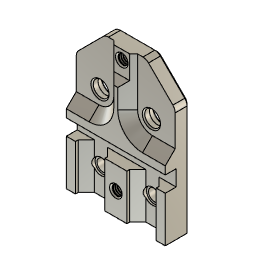
Apollo Yoke Connector P2 [(M)SPPS000000033] v3 (Autodesk Fusion 360 design; units mm, degrees)
Autodesk Fusion 360 part; units mm, degrees
sketch "Sketch1" plane through (0, 0, 0) normal (0, 1, 0) x (1, 0, 0)
  circle A0 centre (0, -5) radius 25
  line L0 (-25, -13.6985) -> (-25, 42)
  line L1 (-25, 42) -> (25, 42)
  line L2 (25, 42) -> (25, -13.6985)
  line L3 (-18, -30) -> (-16.5688, -30)
  line L4 (-8.6985, -30) -> (8.6985, -30)
  line L5 (-23.8284, -16.5269) -> (-11.5269, -28.8284)
  line L6 (11.5269, -28.8284) -> (23.8284, -16.5269)
  arc A1 (-25, -13.6985) -> (-23.8284, -16.5269) centre (-21, -13.6985) ccw
  arc A2 (-11.5269, -28.8284) -> (-8.6985, -30) centre (-8.6985, -26) ccw
  arc A3 (8.6985, -30) -> (11.5269, -28.8284) centre (8.6985, -26) ccw
  arc A4 (23.8284, -16.5269) -> (25, -13.6985) centre (21, -13.6985) ccw
  dimension "d13" = 50
  dimension "d103" = 45
  dimension "d104" = 45
  dimension "d105" = 5
  dimension "d106" = 4
  dimension "d107" = 42
  constraint vertical origin A0.centre
  constraint perpendicular L0 L1
  constraint perpendicular L1 L2
  constraint tangent A0 L0
  constraint tangent A0 L2
  constraint horizontal L1
  constraint horizontal L3
  constraint parallel L3 L4
  constraint tangent A0 L5
  constraint tangent A0 L6
  constraint tangent A0 L4
  constraint tangent L5 A1
  constraint tangent L0 A1
  constraint coincident L3.end L4
  constraint tangent L5 A2
  constraint tangent L4 A2
  constraint equal A1 A2
  constraint tangent L4 A3
  constraint tangent L6 A3
  constraint equal A1 A3
  constraint tangent L6 A4
  constraint tangent L2 A4
  constraint equal A1 A4
  measures "d13" diameter of A0
  measures "d103" angle of L0 L5
  measures "d104" angle of L2 L6
  measures "d105" distance of origin A0.centre
  measures "d106" radius of A1
  measures "d107" distance of origin L1
extrude "Extrude1" add sketch "Sketch1" along normal blind 12
sketch "Sketch2" plane through (0, 0, 0) normal (0, -1, 0) x (1, 0, 0)
  circle A0 centre (-13, -22) radius 8
  circle A1 centre (-13, -22) radius 7.4
  circle A2 centre (13, -22) radius 7.4
  circle A3 centre (13, -22) radius 8
  line L0 (-25, 13.6985) -> (-25, -42)
  line L1 (25, -42) -> (25, 13.6985)
  line L2 (-20.4, -14.6) -> (-20.4, -62.0021)
  line L3 (-5.6, -14.6) -> (-5.6, -62)
  line L4 (5.6, -14.6) -> (5.6, -62.0014)
  line L5 (20.4, -14.6) -> (20.4, -62)
  line L6 (-20.4, -14.6) -> (-5.6, -14.6)
  line L7 (5.6, -14.6) -> (20.4, -14.6)
  line L8 (-15.9, -14.6) -> (-20.4, -19.1)
  line L9 (-10.1, -14.6) -> (-5.6, -19.1)
  line L10 (5.6, -19.1) -> (10.1, -14.6)
  line L11 (15.9, -14.6) -> (20.4, -19.1)
  arc A4 (-23.8284, 16.5269) -> (-25, 13.6985) centre (-21, 13.6985) ccw
  arc A5 (25, 13.6985) -> (23.8284, 16.5269) centre (21, 13.6985) ccw
  line L12 (23.8284, 16.5269) -> (11.5269, 28.8284)
  arc A6 (11.5269, 28.8284) -> (8.6985, 30) centre (8.6985, 26) ccw
  line L13 (8.6985, 30) -> (-8.6985, 30)
  arc A7 (-8.6985, 30) -> (-11.5269, 28.8284) centre (-8.6985, 26) ccw
  line L14 (-11.5269, 28.8284) -> (-23.8284, 16.5269)
  line L15 (-25, -42) -> (25, -42)
  dimension "d36" = 16
  dimension "d37" = 16
  dimension "d38" = 26
  dimension "d7" = 13
  dimension "d8" = 22
  dimension "d9" = 14.8
  dimension "d10" = 14.8
  dimension "d95" = 4.5
  dimension "d96" = 4.5
  dimension "d97" = 4.5
  dimension "d98" = 4.5
  dimension "d99" = 4.5
  dimension "d100" = 4.5
  dimension "d101" = 4.5
  dimension "d102" = 4.5
  constraint concentric A0 A1
  constraint concentric A2 A3
  constraint horizontal A2.centre A0.centre
  constraint tangent A1 L2
  constraint tangent A1 L3
  constraint tangent A2 L4
  constraint tangent A2 L5
  constraint horizontal L7
  constraint tangent A1 L6
  constraint tangent A2 L7
  constraint horizontal L6
  constraint vertical L2
  constraint vertical L3
  constraint vertical L4
  constraint vertical L5
  constraint coincident L6 L8.start
  constraint coincident L2 L8.end
  constraint coincident L6 L9.start
  constraint coincident L3 L9.end
  constraint coincident L4 L10.start
  constraint coincident L7 L10.end
  constraint coincident L7 L11.start
  constraint coincident L5 L11.end
  measures "d36" diameter of A0
  measures "d37" diameter of A3
  measures "d38" distance of A0.centre A2.centre
  measures "d7" horizontal distance of origin A0.centre
  measures "d8" vertical distance of origin A0.centre
  measures "d9" diameter of A1
  measures "d10" diameter of A2
  measures "d95" distance of L8.start L2.start
  measures "d96" distance of L8.end L2.start
  measures "d97" distance of L9.start L3.start
  measures "d98" distance of L9.end L3.start
  measures "d99" distance of L10.start L4.start
  measures "d100" distance of L10.end L4.start
  measures "d101" distance of L11.start L5.start
  measures "d102" distance of L11.end L5.start
extrude "Extrude2" cut sketch "Sketch2" against normal blind 5.5 contours A0 A1 L3 L6 L9 | A0 L3 L6 | A0 L2 L3 L15 | A0 A1 L2 L3 | A0 L6 | A1 L3 L9 | A1 L8 L9 | A0 A1 L2 L6 L8 | A0 L2 L6 | A1 L6 L9 | A1 L9 | A1 L2 L8 | A3 L4 L5 L15 | A1 L6 L8 | A1 L8 | A2 A3 L4 L5 | A3 L4 L7 | A2 A3 L4 L7 L10 | A2 L4 L10 | A2 L10 L11 | A3 L7 | A2 L5 L11 | A2 L10 | A3 L5 L7 | A2 A3 L5 L7 L11 | A2 L7 L10 | A2 L11 | A2 L7 L11
sketch "Sketch3" plane through (0, 0, 0) normal (0, -1, 0) x (1, 0, 0)
  circle A0 centre (0, 5) radius 3
  line L0 (-30.7422, 30.6869) -> (25.9608, 30.6869)
  line L1 (25.9608, 30.6869) -> (25.9608, -2)
  line L2 (25.9608, -2) -> (-30.7422, -2)
  line L3 (-30.7422, -2) -> (-30.7422, 30.6869)
  line L4 (25, -42) -> (25, 13.6985)
  line L5 (-25, 13.6985) -> (-25, -42)
  circle A1 centre (-13, 5) radius 4
  circle A2 centre (13, 5) radius 4
  line L6 (-6, 34) -> (-6, -5)
  line L7 (6, 33) -> (6, -5)
  line L8 (5.6, -42) -> (5.6, -14.6)
  line L9 (5.6, -14.6) -> (9.9603, -14.6)
  line L10 (20.4, -14.6) -> (20.4, -42)
  line L11 (-20.4, -42) -> (-20.4, -14.6)
  line L12 (-20.4, -14.6) -> (-16.0397, -14.6)
  arc A3 (25, 13.6985) -> (23.8284, 16.5269) centre (21, 13.6985) ccw
  line L13 (23.8284, 16.5269) -> (11.5269, 28.8284)
  arc A4 (11.5269, 28.8284) -> (8.6985, 30) centre (8.6985, 26) ccw
  line L14 (8.6985, 30) -> (-8.6985, 30)
  arc A5 (-8.6985, 30) -> (-11.5269, 28.8284) centre (-8.6985, 26) ccw
  line L15 (-11.5269, 28.8284) -> (-23.8284, 16.5269)
  arc A6 (-23.8284, 16.5269) -> (-25, 13.6985) centre (-21, 13.6985) ccw
  line L16 (-5.6, -42) -> (5.6, -42)
  line L17 (20.4, -42) -> (25, -42)
  line L18 (-25, -42) -> (-20.4, -42)
  arc A7 (16.0397, -14.6) -> (9.9603, -14.6) centre (13, -22) ccw
  line L19 (16.0397, -14.6) -> (20.4, -14.6)
  arc A8 (-9.9603, -14.6) -> (-16.0397, -14.6) centre (-13, -22) ccw
  line L20 (-9.9603, -14.6) -> (-5.6, -14.6)
  line L21 (-5.6, -14.6) -> (-5.6, -42)
  dimension "d18" = 6
  dimension "d58" = 5
  dimension "d63" = 7
  dimension "d67" = 8
  dimension "d68" = 8
  dimension "d69" = 26
  dimension "d70" = 13
  dimension "d82" = 7
  dimension "d83" = 7
  constraint horizontal L0
  constraint vertical L1
  constraint horizontal L2
  constraint vertical L3
  constraint vertical origin A0.centre
  constraint horizontal A0.centre A1.centre
  constraint horizontal A0.centre A2.centre
  constraint vertical L6
  constraint perpendicular L2 L7
  measures "d18" diameter of A0
  measures "d58" vertical distance of origin A0.centre
  measures "d63" distance of A0.centre L2
  measures "d67" diameter of A1
  measures "d68" diameter of A2
  measures "d69" horizontal distance of A1.centre A2.centre
  measures "d70" distance of A0.centre A1.centre
  measures "d82" distance of A2.centre L7
  measures "d83" distance of A1.centre L6
sketch "Sketch10" plane through (0, 12, 0) normal (0, 1, 0) x (-1, 0, 0)
  line L0 (-25, 13.6985) -> (-25, -42)
  line L1 (25, -42) -> (25, 13.6985)
  circle A0 centre (0, 5) radius 3
  arc A1 (25, 13.6985) -> (23.8284, 16.5269) centre (21, 13.6985) ccw
  line L2 (23.8284, 16.5269) -> (11.5269, 28.8284)
  arc A2 (11.5269, 28.8284) -> (8.6985, 30) centre (8.6985, 26) ccw
  line L3 (8.6985, 30) -> (-8.6985, 30)
  arc A3 (-8.6985, 30) -> (-11.5269, 28.8284) centre (-8.6985, 26) ccw
  line L4 (-11.5269, 28.8284) -> (-23.8284, 16.5269)
  arc A4 (-23.8284, 16.5269) -> (-25, 13.6985) centre (-21, 13.6985) ccw
  line L5 (-25, -42) -> (25, -42)
  dimension "d84" = 6
  measures "d84" diameter of A0
hole "Hole1" at (0, 12, 5) direction (0, -1, 0) diameter 5.035 depth 9 tip angle 118 countersink diameter 6.82 countersink angle 90
thread "Thread3" "ISO Metric profile 6.0 M6x1 6H" major diameter 6.147 minor diameter 5.035 pitch 1 angle 60 modelled right hand crest width 0.2748 on face at (0.1255, 8.405, 7.5144) crest through (0, 10.8575, 7.5175)
extrude "Extrude8" cut sketch "Sketch3" against normal blind 13 contours A1 | A2
extrude "Extrude9" cut sketch "Sketch3" against normal blind 5 contours L2 L5 L6 L14 A5 L15 A6 | L2 L4 L7 A3 L13 A4 L14
fillet "Fillet1" radius 7.5 2 edges at (6, 2.5, -2) (-6, 2.5, -2)
chamfer "Chamfer9" distance 5 angle 45 6 edges at (8.1967, 0, 0.1967) (6, 0, 17.75) (19.25, 0, -2) (-8.1967, 0, 0.1967) (-19.25, 0, -2) (-6, 0, 17.75)
sketch "Sketch6" plane through (0, 0, 0) normal (0, -1, 0) x (1, 0, 0)
  circle A0 centre (0, 25.3) radius 3
  arc A1 (5.1904, 29.0462) -> (-5.1904, 29.0462) centre (0, 5) ccw
  line L0 (-5.1904, 14.3) -> (5.1904, 14.3)
  line L1 (0, 14.3) -> (0, 29.6)
  line L2 (-5.1904, 29.0462) -> (-5.1904, 14.3)
  line L3 (5.1904, 14.3) -> (5.1904, 29.0462)
  line L4 (-24.4, 5) -> (-24.4, -2)
  line L5 (13, -2) -> (24.4, -2)
  line L6 (24.4, -2) -> (24.4, 5)
  arc A2 (24.4, 5) -> (6, 28.6508) centre (0, 5) ccw
  circle A3 centre (-13, 5) radius 4
  circle A4 centre (13, 5) radius 4
  line L7 (6, 28.6508) -> (6, 5)
  arc A5 (6, 5) -> (13, -2) centre (13, 5) ccw
  arc A6 (-6, 28.6508) -> (-24.4, 5) centre (0, 5) ccw
  line L8 (-24.4, -2) -> (-13, -2)
  arc A7 (-13, -2) -> (-6, 5) centre (-13, 5) ccw
  line L9 (-6, 5) -> (-6, 28.6508)
  line L10 (-6, 32.0092) -> (6, 32.0092)
  line L11 (6, 32.0092) -> (6, 18.3)
  line L12 (6, 18.3) -> (-6, 18.3)
  line L13 (-6, 18.3) -> (-6, 32.0092)
  line L14 (-13.5, -7) -> (-25, -7)
  line L15 (-25, -7) -> (-25, -42)
  line L16 (-25, -42) -> (-20.4, -42)
  line L17 (-20.4, -42) -> (-20.4, -14.6)
  line L18 (-20.4, -14.6) -> (-16.0397, -14.6)
  line L19 (-5.6, -14.6) -> (-5.6, -42)
  line L20 (-5.6, -42) -> (5.6, -42)
  line L21 (5.6, -42) -> (5.6, -14.6)
  line L22 (5.6, -14.6) -> (9.9603, -14.6)
  line L23 (20.4, -14.6) -> (20.4, -42)
  line L24 (20.4, -42) -> (25, -42)
  line L25 (25, -42) -> (25, -7)
  line L26 (25, -7) -> (13.5, -7)
  arc A8 (1, 5.5) -> (13.5, -7) centre (13.5, 5.5) ccw
  line L27 (1, 5.5) -> (1, 30)
  line L28 (1, 30) -> (-1, 30)
  line L29 (-1, 30) -> (-1, 5.5)
  arc A9 (-13.5, -7) -> (-1, 5.5) centre (-13.5, 5.5) ccw
  arc A10 (-9.9603, -14.6) -> (-16.0397, -14.6) centre (-13, -22) ccw
  line L30 (-9.9603, -14.6) -> (-5.6, -14.6)
  arc A11 (16.0397, -14.6) -> (9.9603, -14.6) centre (13, -22) ccw
  line L31 (16.0397, -14.6) -> (20.4, -14.6)
  dimension "d45" = 6
  dimension "d61" = 11
  dimension "d89" = 7
  constraint midpoint L0 L1.start
  constraint midpoint A1 L1.end
  constraint coincident A0.centre L1
  constraint horizontal L10
  constraint vertical L11
  constraint horizontal L12
  constraint vertical L13
  constraint coincident L7 L11.end
  measures "d45" diameter of A0
  measures "d61" distance of A0.centre L0
  measures "d89" distance of A0.centre L12
extrude "Extrude11" cut sketch "Sketch6" against normal blind 3 contours A0 L27 | A0 A1 L3 L12 L27 | A0 L1 L27 | A0 A1 L1 L27 | A0 L1 L12 L27 | A0 L1 L29 | A0 A1 L1 L29 | A1 L2 L3 L7 L9 L10 L11 L12 L13 L27 L28 L29 | A1 L27 L28 L29 | A0 L1 L12 L29 | A0 L29 | A0 A1 L2 L12 L29
sketch "Sketch11" plane through (0, 3, 0) normal (0, -1, 0) x (1, 0, 0)
  circle A0 centre (0, 25.3) radius 3
  line L0 (-4, 30) -> (-4, 18.3)
  line L1 (-4, 18.3) -> (4, 18.3)
  line L2 (4, 18.3) -> (4, 30)
  line L3 (4, 30) -> (-4, 30)
  dimension "d93" = 6
  constraint vertical origin A0.centre
  measures "d93" diameter of A0
hole "Hole2" at (0, 3, 25.3) direction (0, 1, 0) diameter 5.035 depth 24 tip angle 118 countersink diameter 6.4 countersink angle 90
thread "Thread1" "ISO Metric profile 6.0 M6x1 6H" major diameter 6.147 minor diameter 5.035 pitch 1 angle 60 modelled right hand crest width 0.2748 on face at (0.1255, 6.455, 22.7856) crest through (0, 3.9325, 22.7825)
sketch "Sketch7" plane through (0, 0, 0) normal (0, -1, 0) x (1, 0, 0)
  circle A0 centre (0, -30.5) radius 3
  line L0 (1, 18.3) -> (-1, 18.3)
  line L1 (-1, 18.3) -> (-1, 5.5)
  arc A1 (-13.5, -7) -> (-1, 5.5) centre (-13.5, 5.5) ccw
  line L2 (-13.5, -7) -> (-25, -7)
  line L3 (-25, -7) -> (-25, -42)
  line L4 (-25, -42) -> (-20.4, -42)
  line L5 (-20.4, -42) -> (-20.4, -14.6)
  line L6 (-20.4, -14.6) -> (-16.0397, -14.6)
  line L7 (-5.6, -14.6) -> (-5.6, -42)
  line L8 (-5.6, -42) -> (5.6, -42)
  line L9 (5.6, -42) -> (5.6, -14.6)
  line L10 (5.6, -14.6) -> (9.9603, -14.6)
  line L11 (20.4, -14.6) -> (20.4, -42)
  line L12 (20.4, -42) -> (25, -42)
  line L13 (25, -42) -> (25, -7)
  line L14 (25, -7) -> (13.5, -7)
  arc A2 (1, 5.5) -> (13.5, -7) centre (13.5, 5.5) ccw
  line L15 (1, 5.5) -> (1, 18.3)
  arc A3 (-9.9603, -14.6) -> (-16.0397, -14.6) centre (-13, -22) ccw
  line L16 (-9.9603, -14.6) -> (-5.6, -14.6)
  arc A4 (16.0397, -14.6) -> (9.9603, -14.6) centre (13, -22) ccw
  line L17 (16.0397, -14.6) -> (20.4, -14.6)
  dimension "d52" = 6
  dimension "d114" = 11.5
  constraint vertical origin A0.centre
  measures "d52" diameter of A0
  measures "d114" distance of A0.centre L8
hole "Hole3" at (0, 0, -30.5) direction (0, 1, 0) diameter 5.035 depth 13 tip angle 118 countersink diameter 6.4 countersink angle 90
thread "Thread2" "ISO Metric profile 6.0 M6x1 6H" major diameter 6.147 minor diameter 5.035 pitch 1 angle 60 modelled right hand crest width 0.2748 on face at (0.1255, 4.455, -33.0144) crest through (0, 0.9325, -33.0175)
sketch "Sketch9" plane through (0, 12, 0) normal (0, 1, 0) x (-1, 0, 0)
  spline S0 degree 3 poles (-0.4984, -27.4672) (-0.1075, -27.4384) (0.2852, -27.485) (1.0168, -27.7243) (1.3502, -27.9097) (1.9149, -28.3908) (2.1442, -28.6779) (2.4711, -29.3127) (2.5703, -29.6519) (2.6182, -30.2074) (2.6115, -30.4156) (2.549, -30.8208) (2.4946, -31.0166) (2.4172, -31.2036) knots 0 0 0 0 0.117588 0.117588 0.231087 0.231087 0.340498 0.340498 0.445817 0.445817 0.508297 0.508297 0.569249 0.569249 0.569249 0.569249
  arc A0 (-1.0707, -32.7785) -> (2.4172, -31.2036) centre (0, -30.5) ccw
  spline S1 degree 3 poles (-1.0707, -32.7785) (-1.3853, -32.6706) (-1.6753, -32.5012) (-2.1863, -32.0536) (-2.3988, -31.7757) (-2.7141, -31.1427) (-2.809, -30.7914) (-2.8625, -30.0584) (-2.8152, -29.6834) (-2.6249, -29.1021) (-2.524, -28.8866) (-2.2709, -28.4795) (-2.1185, -28.29) (-1.9453, -28.1205) knots 0 0 0 0 0.09977 0.09977 0.203618 0.203618 0.311544 0.311544 0.423544 0.423544 0.494428 0.494428 0.566847 0.566847 0.566847 0.566847
  arc A1 (-0.4984, -27.4672) -> (-1.9453, -28.1205) centre (0, -30.5) ccw
  spline S2 degree 3 poles (-0.4984, 28.3328) (-0.1075, 28.3616) (0.2852, 28.315) (1.0168, 28.0757) (1.3502, 27.8903) (1.9149, 27.4092) (2.1442, 27.1221) (2.4711, 26.4873) (2.5703, 26.1481) (2.6182, 25.5926) (2.6115, 25.3844) (2.549, 24.9792) (2.4946, 24.7834) (2.4172, 24.5964) knots 0 0 0 0 0.117588 0.117588 0.231087 0.231087 0.340498 0.340498 0.445817 0.445817 0.508297 0.508297 0.569249 0.569249 0.569249 0.569249
  spline S3 degree 3 poles (-1.0707, 23.0215) (-1.3853, 23.1294) (-1.6753, 23.2988) (-2.1863, 23.7464) (-2.3988, 24.0243) (-2.7141, 24.6573) (-2.809, 25.0086) (-2.8625, 25.7416) (-2.8152, 26.1166) (-2.6249, 26.6979) (-2.524, 26.9134) (-2.2709, 27.3205) (-2.1185, 27.51) (-1.9453, 27.6795) knots 0 0 0 0 0.09977 0.09977 0.203618 0.203618 0.311544 0.311544 0.423544 0.423544 0.494428 0.494428 0.566847 0.566847 0.566847 0.566847
  arc A2 (-0.4984, 28.3328) -> (-1.9453, 27.6795) centre (0, 25.3) ccw
  circle A3 centre (-13, 5) radius 4
  circle A4 centre (13, 5) radius 4
  circle A5 centre (-13, 5) radius 6
  circle A6 centre (13, 5) radius 6
  arc A7 (-1.0707, 23.0215) -> (2.4172, 24.5964) centre (0, 25.3) ccw
  circle A8 centre (0, 5) radius 3.41
  arc A9 (25, 13.6985) -> (23.8284, 16.5269) centre (21, 13.6985) ccw
  line L0 (23.8284, 16.5269) -> (11.5269, 28.8284)
  arc A10 (11.5269, 28.8284) -> (8.6985, 30) centre (8.6985, 26) ccw
  line L1 (8.6985, 30) -> (-8.6985, 30)
  arc A11 (-8.6985, 30) -> (-11.5269, 28.8284) centre (-8.6985, 26) ccw
  line L2 (-11.5269, 28.8284) -> (-23.8284, 16.5269)
  arc A12 (-23.8284, 16.5269) -> (-25, 13.6985) centre (-21, 13.6985) ccw
  line L3 (-25, 13.6985) -> (-25, -42)
  line L4 (-25, -42) -> (25, -42)
  line L5 (25, -42) -> (25, 13.6985)
  dimension "d77" = 12
  dimension "d78" = 12
  constraint concentric A3 A5
  constraint concentric A4 A6
  measures "d77" diameter of A5
  measures "d78" diameter of A6
extrude "Extrude10" cut sketch "Sketch9" against normal blind 4 contours A5 | A6
sketch "Sketch13" plane through (0, 0, 0) normal (0, -1, 0) x (1, 0, 0)
  circle A0 centre (0, -30.5) radius 3.2
  line L0 (1, 18.3) -> (-1, 18.3)
  line L1 (-1, 18.3) -> (-1, 5.5)
  arc A1 (-13.5, -7) -> (-1, 5.5) centre (-13.5, 5.5) ccw
  line L2 (-13.5, -7) -> (-25, -7)
  line L3 (-25, -7) -> (-25, -42)
  line L4 (-25, -42) -> (-20.4, -42)
  line L5 (-20.4, -42) -> (-20.4, -14.6)
  line L6 (-20.4, -14.6) -> (-16.0397, -14.6)
  line L7 (-5.6, -14.6) -> (-5.6, -42)
  line L8 (-5.6, -42) -> (5.6, -42)
  line L9 (5.6, -42) -> (5.6, -14.6)
  line L10 (5.6, -14.6) -> (9.9603, -14.6)
  line L11 (20.4, -14.6) -> (20.4, -42)
  line L12 (20.4, -42) -> (25, -42)
  line L13 (25, -42) -> (25, -7)
  line L14 (25, -7) -> (13.5, -7)
  arc A2 (1, 5.5) -> (13.5, -7) centre (13.5, 5.5) ccw
  line L15 (1, 5.5) -> (1, 18.3)
  line L16 (-25, -11) -> (25, -11)
  line L17 (25, -11) -> (25, -19)
  line L18 (25, -19) -> (-25, -19)
  line L19 (-25, -19) -> (-25, -11)
  arc A3 (-9.9603, -14.6) -> (-16.0397, -14.6) centre (-13, -22) ccw
  line L20 (-9.9603, -14.6) -> (-5.6, -14.6)
  arc A4 (16.0397, -14.6) -> (9.9603, -14.6) centre (13, -22) ccw
  line L21 (16.0397, -14.6) -> (20.4, -14.6)
  dimension "d118" = 4
  dimension "d119" = 8
  constraint horizontal L16
  constraint vertical L17
  constraint horizontal L18
  constraint vertical L19
  constraint coincident L13 L17.end
  constraint coincident L3 L16.start
  measures "d118" distance of L2 L16
  measures "d119" distance of L16 L18
extrude "Extrude12" cut sketch "Sketch13" against normal up to surface (5.5 mm away) contours L3 L5 L6 L7 L9 L10 L11 L13 L16 L17 L18 L19 A3 L20 A4 L21
chamfer "Chamfer7" distance 0.6 angle 45 4 edges at (9.2707, 5, 3.5535) (-16.7293, 5, 3.5535) (-7.406, 12, 7.1697) (18.594, 12, 7.1697)
chamfer "Chamfer11" distance 1 angle 45 10 edges at (-25, 12, -14.1508) (-24.6955, 12, 15.2292) (-17.6777, 12, 22.6777) (-10.2292, 12, 29.6955) (0, 12, 30) (10.2292, 12, 29.6955) (17.6777, 12, 22.6777) (24.6955, 12, 15.2292) (25, 12, -14.1508) (0, 12, -42)
chamfer "Chamfer12" distance 3 angle 45 1 edges at (0, 0, 18.3)
sketch "Sketch14" plane through (0, 0, -42) normal (0, 0, -1) x (1, 0, 0)
  line L0 (-25, -11) -> (25, -11)
  line L1 (20.4, 0) -> (20.4, -5.5)
  line L2 (20.4, -5.5) -> (5.6, -5.5)
  line L3 (5.6, -5.5) -> (5.6, 0)
  line L4 (-5.6, 0) -> (-5.6, -5.5)
  line L5 (-5.6, -5.5) -> (-20.4, -5.5)
  line L6 (-20.4, -5.5) -> (-20.4, 0)
  circle A0 centre (-13, 2.5) radius 8
  line L7 (-20.4, -1.4137) -> (-15.7271, -6.0866)
  line L8 (-20.3137, -1.5) -> (-14.0283, -1.5) construction
  line L9 (-10.1863, -6) -> (-5.4941, -1.3078)
  line L10 (-10.1863, -6) -> (-3.7889, -6) construction
  circle A1 centre (13, 2.5) radius 8
  line L11 (5.6, -1.4137) -> (10.2729, -6.0866)
  line L12 (15.8137, -6) -> (20.5059, -1.3078)
  line L13 (25, -11) -> (25, 0)
  line L14 (25, 0) -> (20.4, 0)
  line L15 (5.6, 0) -> (-5.6, 0)
  line L16 (-20.4, 0) -> (-25, 0)
  line L17 (-25, 0) -> (-25, -11)
  dimension "d122" = 16
  dimension "d123" = 45
  dimension "d124" = 45
  dimension "d125" = 16
  constraint tangent L5 A0
  constraint horizontal L8
  constraint horizontal L10
  constraint tangent A0 L9
  constraint tangent A0 L7
  constraint coincident L6 L7.start
  constraint coincident L8.start L7
  constraint tangent A1 L12
  constraint tangent A1 L11
  measures "d122" diameter of A0
  measures "d123" angle of L7 L8
  measures "d124" angle of L9 L10
  measures "d125" diameter of A1
extrude "Extrude13" add sketch "Sketch14" against normal up to surface (23 mm away) contours L5 L6 L7 | L1 L2 L12 | L4 L5 L9 | L2 L3 L11
sketch "Sketch15" plane through (0, 12, 0) normal (0, 1, 0) x (-1, 0, 0)
  line L0 (-24, -41) -> (24, -41)
  line L1 (24, -41) -> (24, 13.6985)
  arc A0 (24, 13.6985) -> (23.1213, 15.8198) centre (21, 13.6985) ccw
  line L2 (23.1213, 15.8198) -> (10.8198, 28.1213)
  arc A1 (10.8198, 28.1213) -> (8.6985, 29) centre (8.6985, 26) ccw
  line L3 (8.6985, 29) -> (-8.6985, 29)
  arc A2 (-8.6985, 29) -> (-10.8198, 28.1213) centre (-8.6985, 26) ccw
  line L4 (-10.8198, 28.1213) -> (-23.1213, 15.8198)
  arc A3 (-23.1213, 15.8198) -> (-24, 13.6985) centre (-21, 13.6985) ccw
  line L5 (-24, 13.6985) -> (-24, -41)
  circle A4 centre (-13, 5) radius 6.6
  circle A5 centre (0, 5) radius 3.41
  spline S0 degree 3 poles (-0.4984, 28.3328) (-0.1075, 28.3616) (0.2852, 28.315) (1.0168, 28.0757) (1.3502, 27.8903) (1.9149, 27.4092) (2.1442, 27.1221) (2.4711, 26.4873) (2.5703, 26.1481) (2.6182, 25.5926) (2.6115, 25.3844) (2.549, 24.9792) (2.4946, 24.7834) (2.4172, 24.5964) knots 0 0 0 0 0.117588 0.117588 0.231087 0.231087 0.340498 0.340498 0.445817 0.445817 0.508297 0.508297 0.569249 0.569249 0.569249 0.569249
  arc A6 (-1.0707, 23.0215) -> (2.4172, 24.5964) centre (0, 25.3) ccw
  spline S1 degree 3 poles (-1.0707, 23.0215) (-1.3853, 23.1294) (-1.6753, 23.2988) (-2.1863, 23.7464) (-2.3988, 24.0243) (-2.7141, 24.6573) (-2.809, 25.0086) (-2.8625, 25.7416) (-2.8152, 26.1166) (-2.6249, 26.6979) (-2.524, 26.9134) (-2.2709, 27.3205) (-2.1185, 27.51) (-1.9453, 27.6795) knots 0 0 0 0 0.09977 0.09977 0.203618 0.203618 0.311544 0.311544 0.423544 0.423544 0.494428 0.494428 0.566847 0.566847 0.566847 0.566847
  arc A7 (-0.4984, 28.3328) -> (-1.9453, 27.6795) centre (0, 25.3) ccw
  spline S2 degree 3 poles (-0.4984, -27.4672) (-0.1075, -27.4384) (0.2852, -27.485) (1.0168, -27.7243) (1.3502, -27.9097) (1.9149, -28.3908) (2.1442, -28.6779) (2.4711, -29.3127) (2.5703, -29.6519) (2.6182, -30.2074) (2.6115, -30.4156) (2.549, -30.8208) (2.4946, -31.0166) (2.4172, -31.2036) knots 0 0 0 0 0.117588 0.117588 0.231087 0.231087 0.340498 0.340498 0.445817 0.445817 0.508297 0.508297 0.569249 0.569249 0.569249 0.569249
  arc A8 (-1.0707, -32.7785) -> (2.4172, -31.2036) centre (0, -30.5) ccw
  spline S3 degree 3 poles (-1.0707, -32.7785) (-1.3853, -32.6706) (-1.6753, -32.5012) (-2.1863, -32.0536) (-2.3988, -31.7757) (-2.7141, -31.1427) (-2.809, -30.7914) (-2.8625, -30.0584) (-2.8152, -29.6834) (-2.6249, -29.1021) (-2.524, -28.8866) (-2.2709, -28.4795) (-2.1185, -28.29) (-1.9453, -28.1205) knots 0 0 0 0 0.09977 0.09977 0.203618 0.203618 0.311544 0.311544 0.423544 0.423544 0.494428 0.494428 0.566847 0.566847 0.566847 0.566847
  arc A9 (-0.4984, -27.4672) -> (-1.9453, -28.1205) centre (0, -30.5) ccw
  circle A10 centre (13, 5) radius 6.6
  circle A11 centre (-13, -29) radius 1.5
  circle A12 centre (13, -29) radius 1.5
  line L6 (25, -11) -> (-25, -11)
  dimension "d128" = 3
  dimension "d129" = 3
  dimension "d130" = 26
  dimension "d143" = 18
  dimension "d144" = 13
  constraint horizontal A11.centre A12.centre
  measures "d128" diameter of A11
  measures "d129" diameter of A12
  measures "d130" distance of A11.centre A12.centre
  measures "d143" distance of A12.centre L6
  measures "d144" horizontal distance of A8.centre A12.centre
hole "Hole4" at (13, 12, -29) at (-13, 12, -29) direction (0, -1, 0) diameter 6 depth 7 tip angle 118
sketch "Sketch16" plane through (0, 5.5, 0) normal (0, -1, 0) x (1, 0, 0)
  circle A0 centre (13, -29) radius 3
  circle A1 centre (-13, -29) radius 3
  line L0 (16.3137, -19) -> (25, -19)
  line L1 (25, -19) -> (25, -11)
  line L2 (25, -11) -> (-25, -11)
  line L3 (-25, -11) -> (-25, -19)
  line L4 (-25, -19) -> (-16.3137, -19)
  line L5 (-16.3137, -19) -> (-16.3137, -42)
  line L6 (-16.3137, -42) -> (-9.6863, -42)
  line L7 (-9.6863, -42) -> (-9.6863, -19)
  line L8 (-9.6863, -19) -> (9.6863, -19)
  line L9 (9.6863, -19) -> (9.6863, -42)
  line L10 (9.6863, -42) -> (16.3137, -42)
  line L11 (16.3137, -42) -> (16.3137, -19)
  circle A2 centre (-13, -29) radius 4
  circle A3 centre (13, -29) radius 4
  dimension "d137" = 8
  dimension "d138" = 8
  constraint concentric A1 A2
  constraint concentric A0 A3
  measures "d137" diameter of A2
  measures "d138" diameter of A3
extrude "Extrude14" cut sketch "Sketch16" along normal blind 3 and the other way blind 1 contours L11 A3 | L9 L11 A3 | L9 A3 | L7 A2 | L5 L7 A2 | L5 A2
equation "d7 = d38 / 2"
equation "d70 = d69 / 2"
equation "d96 = d95"
equation "d98 = d97"
equation "d100 = d99"
equation "d102 = d101"
equation "d144 = d130 / 2"
